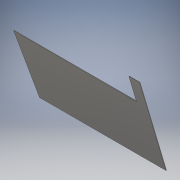
# Autodesk Inventor part: Cabin Side Panel
Saved by Autodesk Inventor 2019 (Build 230136000, 136)
## iProperties
Created: 2019-08-30
Part Number: Cabin Side Panel
Material: Steel, Mild
Document SubType Name: Modeling
Designer: DIBYOJYOTI
Density: 7.85 g/cm^3
Appearance: Semi-Polished
Author: DIBYOJYOTI
Autodesk Inventor part; units mm, degrees
ref_plane "YZ Plane" through (0, 0, 0) normal (1, 0, 0) x (0, 1, 0)
ref_plane "XZ Plane" through (0, 0, 0) normal (0, 1, 0) x (-1, 0, 0)
ref_plane "XY Plane" through (0, 0, 0) normal (0, 0, 1) x (1, 0, 0)
derived "Cabin Wall.ipt"
sketch "Sketch5" plane through (249.6025, 52.3237, -1) normal (0, 0, 1) x (1, 0, 0)
  line L0 (-41.0092, -56.3237) -> (-277.8705, -56.3237)
  line L1 (-90.4064, 61.6763) -> (-41.0092, -56.3237)
  line L2 (-41.0092, -56.3237) -> (-277.8705, -56.3237)
  line L3 (-277.8705, -56.3237) -> (-326.6025, 28.0827)
  line L4 (-277.8705, -56.3237) -> (-326.6025, 28.0827)
  line L5 (-326.6025, 28.0827) -> (-326.6025, 61.6763)
  line L6 (-326.6025, 28.0827) -> (-326.6025, 61.6763)
  line L7 (-326.6025, 61.6763) -> (-90.4064, 61.6763)
  line L8 (-76.3434, 28.0827) -> (-96.3434, 28.0827)
  line L9 (-96.3434, 28.0827) -> (-110.4064, 61.6763)
  line L10 (-326.6025, 61.6763) -> (-90.4064, 61.6763)
  line L11 (-326.6025, 28.0827) -> (-326.6025, 61.6763)
  line L12 (-326.6025, 61.6763) -> (-205.3471, 61.6763)
  line L13 (-326.6025, 28.0827) -> (-279.094, 28.0827) construction
  line L14 (-293.0089, 61.6763) -> (-110.4064, 61.6763)
  line L15 (-133.858, 61.6763) -> (-90.4064, 61.6763)
  line L16 (-326.6025, 28.0827) -> (-96.3434, 28.0827)
  point P0 (-249.6025, -52.3237)
  dimension "d5" = 20
  dimension "d6" = 216.1961
  dimension "d11" = 118
  dimension "d12" = 84.4064
  dimension "d13" = 236.8613
  constraints: 34 end point
  measures "d5" distance of L9.end L1.start
  measures "d6" distance of L5.end L9.end
  measures "d11" vertical distance of L1.start L0.start
  measures "d12" vertical distance of L0.end L3.end
  measures "d13" distance of L0.start L0.end
extrude "Extrusion3" add sketch "Sketch5" against normal blind 1 contours L8 L9 L7 L1
extrude "Extrusion4" add sketch "Sketch5" against normal blind 1 contours L0 L3 L16 L8 L1
body "Solid2"
